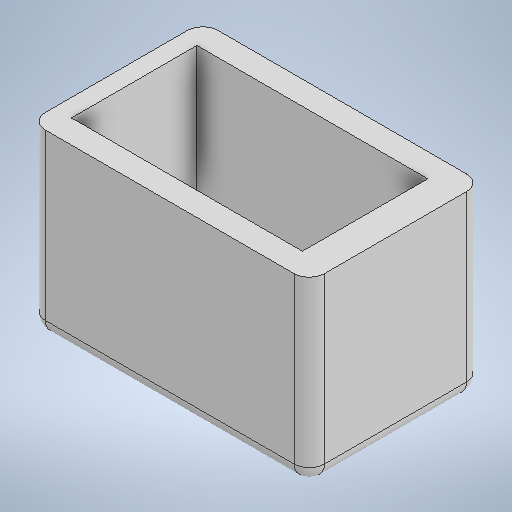
# Autodesk Inventor part: basketlewy
Saved by Autodesk Inventor 2025.3 (Build 293356000, 356)
## iProperties
Created: 2026-04-05
Part Number: basketlewy
Material: Generic
Document SubType Name: Modeling
Designer: ksawe
Density: 1 g/cm^3
Appearance: Default
Author: ksawe
Autodesk Inventor part; units mm, degrees
ref_plane "YZ Plane" through (0, 0, 0) normal (1, 0, 0) x (0, 1, 0)
ref_plane "XZ Plane" through (0, 0, 0) normal (0, 1, 0) x (-1, 0, 0)
ref_plane "XY Plane" through (0, 0, 0) normal (0, 0, 1) x (1, 0, 0)
sketch "Sketch1" plane through (0, 0, 0) normal (0, 1, 0) x (-1, 0, 0)
  line L0 (22.75, -10.36) -> (7.75, -10.36)
  line L1 (7.75, -10.36) -> (-0.1031, 0)
  circle A0 centre (4.34, -10.36) radius 1
  line L2 (22.75, 10.36) -> (7.75, 10.36)
  circle A1 centre (12.64, 0) radius 9.6 construction
  line L3 (22.75, 12.36) -> (22.75, -12.36)
  circle A2 centre (4.34, 10.36) radius 1
  line L4 (7.75, 10.36) -> (-0.1031, 0)
  line L5 (26.25, 17) -> (26.25, -17)
  line L6 (22.75, -12.36) -> (-22.75, -12.36)
  line L7 (22.75, 0) -> (-22.75, 0) construction
  line L8 (26.25, -17) -> (-28.75, -17)
  line L9 (26.25, -17) -> (-28.75, 17) construction
  line L10 (-28.75, -17) -> (26.25, 17) construction
  line L11 (-22.75, 12.36) -> (22.75, 12.36)
  line L12 (-28.75, 17) -> (26.25, 17)
  line L13 (-28.75, -17) -> (-28.75, 17)
  circle A3 centre (-16.36, 10.25) radius 1
  line L14 (-22.75, -12.36) -> (-22.75, 12.36)
  circle A4 centre (-16.36, -10.25) radius 1
  point P0 (0, 0)
  point P1 (-1.25, 0)
  point P2 (0, 0)
  point P3 (22.75, -10.36)
  dimension "d0" = 55
  dimension "d1" = 34
  dimension "d2" = 45.5
  dimension "d3" = 24.72
  dimension "d4" = 2
  dimension "d6" = 18.41
  dimension "d7" = 20.5
  dimension "d8" = 19.2
  dimension "d9" = 10.11
  dimension "d10" = 13
  dimension "d11" = 15
  dimension "d12" = 3.5
  dimension "d13" = 2
  dimension "d14" = 3.41
  dimension "d66" = 20.7
  constraints: 30 end point, 5 centre point, 5 midpoint, 4 parallel, 4 symmetric about line, 3 horizontal, 3 point on line, 2 coincident, 2 perpendicular, 1 equal radius, 1 horizontal alignment, 3 other
  measures "d0" distance of L9.end L5.start
  measures "d1" distance of L8.end L9.end
  measures "d2" distance of L11.start L3.start
  measures "d3" distance of L6.end L11.start
  measures "d4" diameter of A2
  measures "d6" distance from line of L3 A2.centre
  measures "d7" distance of A3.centre A4.centre
  measures "d8" diameter of A1
  measures "d9" distance from line of L3 A1.centre
  measures "d10" distance of L2.end L1.end
  measures "d11" distance of L2.start L2.end
  measures "d12" distance between parallel lines of L5 L3
  measures "d13" distance between parallel lines of L11 L2
  measures "d14" distance of A2.centre L2.end
  measures "d66" horizontal distance of A3.centre A2.centre
extrude "Extrusion1" add sketch "Sketch1" along normal mid plane 1 contours L3 L6 L14 L11 L2 L4 L1 L0 | L5 L8 L13 L12
extrude "Extrusion2" add sketch "Sketch1" along normal blind 35 contours L5 L8 L13 L12
fillet "Fillet1" radius 3 8 edges at (1.25, -0.5, -17) (28.75, -0.5, 0) (1.25, -0.5, 17) (-26.25, -0.5, 0) (28.75, 17.25, -17) (28.75, 17.25, 17) (-26.25, 17.25, 17) (-26.25, 17.25, -17)
sketch "Sketch5" plane through (25.75, 2.5, -17) normal (0, 0, -1) x (-1, 0, 0)
  circle A0 centre (6, 4.5) radius 1.5
  line L0 (0, 0) -> (0, 32.5) projected
  line L1 (49, 0) -> (0, 0) projected
  circle A1 centre (6, 15.5) radius 1.5
  circle A2 centre (6, 26.5) radius 1.5
  circle A3 centre (22, 4.5) radius 1.5
  circle A4 centre (22, 15.5) radius 1.5
  circle A5 centre (22, 26.5) radius 1.5
  point P0 (25.75, -2.5)
  dimension "d47" = 3
  dimension "d48" = 6
  dimension "d49" = 4.5
  dimension "d52" = 11
  dimension "d55" = 16
  constraints: 6 centre point, 1 horizontal, 1 vertical, 10 other
  measures "d47" diameter of A0
  measures "d48" distance from line of L0 A0.centre
  measures "d49" distance from line of L1 A0.centre
  measures "d52" distance of A0.centre A1.centre
  measures "d55" distance of A0.centre A3.centre
hole "Hole2" at (19.75, 7, -17) at (19.75, 18, -17) at (3.75, 18, -17) at (3.75, 7, -17) at (19.75, 29, -17) at (3.75, 29, -17) direction (0, 0, 1) diameter 2.459 depth 3 tip angle 118 counterbore diameter 3.9 counterbore depth 1.8 thread size "M3x0.5" class "6H" standard "ISO Metric profile"
body "Solid1"
